Autodesk Fusion 360 part; units mm, degrees
note: some values were not read from the file. Set by a fixed rule: which sketch regions a step uses.
(part 2 of 2)
sketch "Esquisse1 (2)" plane through (0, 0, -35) normal (0, 0, -1) x (1, 0, 0) in component "Component"
  circle A0 centre (290, 50) radius 1.7
  circle A1 centre (10, 10) radius 1.7
  circle A2 centre (80, 90) radius 1.7
  circle A3 centre (150, 10) radius 1.7
  circle A4 centre (220, 90) radius 1.7
  line L0 (282, 72) -> (282, 28)
  arc A5 (272, 18) -> (282, 28) centre (272, 28) ccw
  line L1 (272, 18) -> (28, 18)
  arc A6 (18, 28) -> (28, 18) centre (28, 28) ccw
  line L2 (18, 28) -> (18, 72)
  arc A7 (28, 82) -> (18, 72) centre (28, 72) ccw
  line L3 (28, 82) -> (272, 82)
  arc A8 (282, 72) -> (272, 82) centre (272, 72) ccw
  circle A9 centre (10, 50) radius 1.7
  circle A10 centre (80, 10) radius 1.7
  circle A11 centre (290, 90) radius 1.7
  circle A12 centre (220, 10) radius 1.7
  circle A13 centre (150, 90) radius 1.7
  circle A14 centre (10, 90) radius 1.7
  circle A15 centre (290, 10) radius 1.7
  line L4 (290, 100) -> (10, 100)
  arc A16 (10, 100) -> (0, 90) centre (10, 90) ccw
  line L5 (0, 90) -> (0, 10)
  arc A17 (0, 10) -> (10, 0) centre (10, 10) ccw
  line L6 (10, 0) -> (290, 0)
  arc A18 (290, 0) -> (300, 10) centre (290, 10) ccw
  line L7 (300, 10) -> (300, 90)
  arc A19 (300, 90) -> (290, 100) centre (290, 90) ccw
  line L8 (12.75, 91.587713) -> (10, 93.175426)
  line L9 (10, 93.175426) -> (7.25, 91.587713)
  line L10 (7.25, 91.587713) -> (7.25, 88.412287)
  line L11 (7.25, 88.412287) -> (10, 86.824574)
  line L12 (10, 86.824574) -> (12.75, 88.412287)
  line L13 (12.75, 88.412287) -> (12.75, 91.587713)
  line L14 (80, 93.175426) -> (77.25, 91.587713)
  line L15 (77.25, 91.587713) -> (77.25, 88.412287)
  line L16 (77.25, 88.412287) -> (80, 86.824574)
  line L17 (80, 86.824574) -> (82.75, 88.412287)
  line L18 (82.75, 88.412287) -> (82.75, 91.587713)
  line L19 (82.75, 91.587713) -> (80, 93.175426)
  line L20 (150, 93.175426) -> (147.25, 91.587713)
  line L21 (147.25, 91.587713) -> (147.25, 88.412287)
  line L22 (147.25, 88.412287) -> (150, 86.824574)
  line L23 (150, 86.824574) -> (152.75, 88.412287)
  line L24 (152.75, 88.412287) -> (152.75, 91.587713)
  line L25 (152.75, 91.587713) -> (150, 93.175426)
  line L26 (222.75, 88.412287) -> (222.75, 91.587713)
  line L27 (222.75, 91.587713) -> (220, 93.175426)
  line L28 (220, 93.175426) -> (217.25, 91.587713)
  line L29 (217.25, 91.587713) -> (217.25, 88.412287)
  line L30 (217.25, 88.412287) -> (220, 86.824574)
  line L31 (220, 86.824574) -> (222.75, 88.412287)
  line L32 (290, 86.824574) -> (292.75, 88.412287)
  line L33 (292.75, 88.412287) -> (292.75, 91.587713)
  line L34 (292.75, 91.587713) -> (290, 93.175426)
  line L35 (290, 93.175426) -> (287.25, 91.587713)
  line L36 (287.25, 91.587713) -> (287.25, 88.412287)
  line L37 (287.25, 88.412287) -> (290, 86.824574)
  line L38 (292.75, 51.587713) -> (290, 53.175426)
  line L39 (290, 53.175426) -> (287.25, 51.587713)
  line L40 (287.25, 51.587713) -> (287.25, 48.412287)
  line L41 (287.25, 48.412287) -> (290, 46.824574)
  line L42 (290, 46.824574) -> (292.75, 48.412287)
  line L43 (292.75, 48.412287) -> (292.75, 51.587713)
  line L44 (292.75, 8.412287) -> (292.75, 11.587713)
  line L45 (292.75, 11.587713) -> (290, 13.175426)
  line L46 (290, 13.175426) -> (287.25, 11.587713)
  line L47 (287.25, 11.587713) -> (287.25, 8.412287)
  line L48 (287.25, 8.412287) -> (290, 6.824574)
  line L49 (290, 6.824574) -> (292.75, 8.412287)
  line L50 (222.75, 8.412287) -> (222.75, 11.587713)
  line L51 (222.75, 11.587713) -> (220, 13.175426)
  line L52 (220, 13.175426) -> (217.25, 11.587713)
  line L53 (217.25, 11.587713) -> (217.25, 8.412287)
  line L54 (217.25, 8.412287) -> (220, 6.824574)
  line L55 (220, 6.824574) -> (222.75, 8.412287)
  line L56 (152.75, 8.412287) -> (152.75, 11.587713)
  line L57 (152.75, 11.587713) -> (150, 13.175426)
  line L58 (150, 13.175426) -> (147.25, 11.587713)
  line L59 (147.25, 11.587713) -> (147.25, 8.412287)
  line L60 (147.25, 8.412287) -> (150, 6.824574)
  line L61 (150, 6.824574) -> (152.75, 8.412287)
  line L62 (82.75, 8.412287) -> (82.75, 11.587713)
  line L63 (82.75, 11.587713) -> (80, 13.175426)
  line L64 (80, 13.175426) -> (77.25, 11.587713)
  line L65 (77.25, 11.587713) -> (77.25, 8.412287)
  line L66 (77.25, 8.412287) -> (80, 6.824574)
  line L67 (80, 6.824574) -> (82.75, 8.412287)
  line L68 (12.75, 11.587713) -> (10, 13.175426)
  line L69 (10, 13.175426) -> (7.25, 11.587713)
  line L70 (7.25, 11.587713) -> (7.25, 8.412287)
  line L71 (7.25, 8.412287) -> (10, 6.824574)
  line L72 (10, 6.824574) -> (12.75, 8.412287)
  line L73 (12.75, 8.412287) -> (12.75, 11.587713)
  line L74 (12.75, 48.412287) -> (12.75, 51.587713)
  line L75 (12.75, 51.587713) -> (10, 53.175426)
  line L76 (10, 53.175426) -> (7.25, 51.587713)
  line L77 (7.25, 51.587713) -> (7.25, 48.412287)
  line L78 (7.25, 48.412287) -> (10, 46.824574)
  line L79 (10, 46.824574) -> (12.75, 48.412287)
  circle A20 centre (158.099746, 49.935862) radius 1.7
  circle A21 centre (141.900254, 50.064138) radius 1.7
  line L80 (158.099746, 49.935862) -> (141.900254, 50.064138) construction
  line L81 (0, 90) -> (0, 10) construction
  line L82 (300, 10) -> (300, 90) construction
  point P0 (10, 90)
  point P1 (80, 90)
  point P2 (150, 90)
  point P3 (220, 90)
  point P4 (290, 90)
  point P5 (290, 50)
  point P6 (290, 10)
  point P7 (220, 10)
  point P8 (150, 10)
  point P9 (80, 10)
  point P10 (10, 10)
  point P11 (10, 50)
  point P12 (158.099746, 49.935862)
  point P13 (141.900254, 50.064138)
  point P14 (150, 50)
  point P15 (0, 90)
  point P16 (290, 100)
  dimension "d71" = 5.5
  dimension "d72" = 5.5
  dimension "d73" = 5.5
  dimension "d78" = 5.5
  dimension "d79" = 5.5
  dimension "d80" = 5.5
  dimension "d81" = 5.5
  dimension "d82" = 5.5
  dimension "d83" = 5.5
  dimension "d84" = 5.5
  dimension "d85" = 5.5
  dimension "d86" = 5.5
  dimension "d92" = 3.4
  dimension "d93" = 3.4
  dimension "d94" = 16.2
  dimension "d122" = 150
  dimension "d123" = 300
  dimension "d124" = 100
  dimension "d125" = 50
  constraint coincident P0 A14.centre
  constraint vertical L13
  constraint coincident P1 A2.centre
  constraint coincident P2 A13.centre
  constraint vertical L18
  constraint vertical L24
  constraint coincident P3 A4.centre
  constraint coincident P4 A11.centre
  constraint coincident P5 A0.centre
  constraint coincident P6 A15.centre
  constraint coincident P7 A12.centre
  constraint coincident P8 A3.centre
  constraint coincident P9 A10.centre
  constraint coincident P10 A1.centre
  constraint coincident P11 A9.centre
  constraint vertical L26
  constraint vertical L33
  constraint vertical L43
  constraint vertical L44
  constraint vertical L50
  constraint vertical L56
  constraint vertical L62
  constraint vertical L73
  constraint vertical L74
  constraint midpoint L80 P14
  measures "d78" distance of L26 L29
  measures "d79" distance of L33 L36
  measures "d80" distance of L40 L43
  measures "d81" distance of L44 L47
  measures "d82" distance of L50 L53
  measures "d83" distance of L56 L59
  measures "d84" distance of L62 L65
  measures "d85" distance of L70 L73
  measures "d86" distance of L74 L77
  measures "d92" diameter of A20
  measures "d93" diameter of A21
  measures "d122" distance of P14 L81
  measures "d123" distance of P15 L82
  measures "d124" distance of L6 P16
  measures "d125" distance of L4 P14
extrude "Extrusion4" cut sketch "Esquisse1 (2)" against normal blind 25 contours A0 | A1 | A2 | A3 | A4 | A9 | A10 | A11 | A12 | A13 | A14 | A15 | L8 L9 L10 L11 L12 L13 | L14 L15 L16 L17 L18 L19 | L20 L21 L22 L23 L24 L25 | L26 L27 L28 L29 L30 L31 | L32 L33 L34 L35 L36 L37 | L38 L39 L40 L41 L42 L43 | L44 L45 L46 L47 L48 L49 | L50 L51 L52 L53 L54 L55 | L56 L57 L58 L59 L60 L61 | L62 L63 L64 L65 L66 L67 | L68 L69 L70 L71 L72 L73 | L74 L75 L76 L77 L78 L79 picked at (289.075398, 49.754133) picked at (10.073289, 9.513757) picked at (80.368027, 90.490748) picked at (150.541491, 10.001887) picked at (218.751887, 89.832972) picked at (10.353311, 50.777094) picked at (80.199585, 10.503371) picked at (289.075398, 89.754133) picked at (218.891842, 10.167028) picked at (150.541491, 90.001887) picked at (9.024266, 90.469889) picked at (291.077216, 10.245867) picked at (11.2, 87.921539) picked at (78.8, 87.921539) picked at (151.2, 92.078461) picked at (218.8, 87.921539) picked at (291.2, 87.921539) picked at (291.2, 52.078461) picked at (292.4, 10) picked at (222.4, 10) picked at (151.2, 7.921539) picked at (81.2, 7.921539) picked at (12.4, 10) picked at (12.4, 50) bodies 2 in component "Component"
extrude "Extrusion3" add sketch "Esquisse1 (2)" along normal blind 5 contours L0 A5 L1 A6 L2 A7 L3 A8 | L4 A16 L5 A17 L6 A18 L7 A19 | A20 | A21 picked at (65.400085, 50.021379) picked at (38.416667, 8.804096) picked at (156.991588, 49.768834) picked at (142.441745, 50.066024) bodies 2 in component "Component"
extrude "Extrusion5'" add 1 faces at (55.75, -50.529238, -40) along direction (0, 0, -1) blind 1 on bodies 2 bodies 2 in component "Component"
extrude "Extrusion6'" cut sketch "Esquisse1 (2)" along normal blind 10 contours A20 | A21 picked at (156.991588, 49.768834) picked at (142.441745, 50.066024) bodies 2 in component "Component"
sketch "Esquisse3 (2)" plane through (0, 0, -41) normal (0, 0, -1) x (1, 0, 0) in component "Component"
  circle A0 centre (141.900254, 50.064138) radius 1.7
  circle A1 centre (158.099746, 49.935862) radius 1.7
  line L0 (12.75, 11.587713) -> (12.75, 8.412287)
  line L1 (12.75, 8.412287) -> (10, 6.824574)
  line L2 (10, 6.824574) -> (7.25, 8.412287)
  line L3 (7.25, 8.412287) -> (7.25, 11.587713)
  line L4 (7.25, 11.587713) -> (10, 13.175426)
  line L5 (10, 13.175426) -> (12.75, 11.587713)
  line L6 (12.75, 48.412287) -> (10, 46.824574)
  line L7 (10, 46.824574) -> (7.25, 48.412287)
  line L8 (7.25, 48.412287) -> (7.25, 51.587713)
  line L9 (7.25, 51.587713) -> (10, 53.175426)
  line L10 (10, 53.175426) -> (12.75, 51.587713)
  line L11 (12.75, 51.587713) -> (12.75, 48.412287)
  line L12 (222.75, 88.412287) -> (220, 86.824574)
  line L13 (220, 86.824574) -> (217.25, 88.412287)
  line L14 (217.25, 88.412287) -> (217.25, 91.587713)
  line L15 (217.25, 91.587713) -> (220, 93.175426)
  line L16 (220, 93.175426) -> (222.75, 91.587713)
  line L17 (222.75, 91.587713) -> (222.75, 88.412287)
  line L18 (12.75, 91.587713) -> (12.75, 88.412287)
  line L19 (12.75, 88.412287) -> (10, 86.824574)
  line L20 (10, 86.824574) -> (7.25, 88.412287)
  line L21 (7.25, 88.412287) -> (7.25, 91.587713)
  line L22 (7.25, 91.587713) -> (10, 93.175426)
  line L23 (10, 93.175426) -> (12.75, 91.587713)
  line L24 (150, 93.175426) -> (152.75, 91.587713)
  line L25 (152.75, 91.587713) -> (152.75, 88.412287)
  line L26 (152.75, 88.412287) -> (150, 86.824574)
  line L27 (150, 86.824574) -> (147.25, 88.412287)
  line L28 (147.25, 88.412287) -> (147.25, 91.587713)
  line L29 (147.25, 91.587713) -> (150, 93.175426)
  line L30 (290, 86.824574) -> (287.25, 88.412287)
  line L31 (287.25, 88.412287) -> (287.25, 91.587713)
  line L32 (287.25, 91.587713) -> (290, 93.175426)
  line L33 (290, 93.175426) -> (292.75, 91.587713)
  line L34 (292.75, 91.587713) -> (292.75, 88.412287)
  line L35 (292.75, 88.412287) -> (290, 86.824574)
  line L36 (222.75, 8.412287) -> (220, 6.824574)
  line L37 (220, 6.824574) -> (217.25, 8.412287)
  line L38 (217.25, 8.412287) -> (217.25, 11.587713)
  line L39 (217.25, 11.587713) -> (220, 13.175426)
  line L40 (220, 13.175426) -> (222.75, 11.587713)
  line L41 (222.75, 11.587713) -> (222.75, 8.412287)
  line L42 (80, 93.175426) -> (82.75, 91.587713)
  line L43 (82.75, 91.587713) -> (82.75, 88.412287)
  line L44 (82.75, 88.412287) -> (80, 86.824574)
  line L45 (80, 86.824574) -> (77.25, 88.412287)
  line L46 (77.25, 88.412287) -> (77.25, 91.587713)
  line L47 (77.25, 91.587713) -> (80, 93.175426)
  line L48 (292.75, 51.587713) -> (292.75, 48.412287)
  line L49 (292.75, 48.412287) -> (290, 46.824574)
  line L50 (290, 46.824574) -> (287.25, 48.412287)
  line L51 (287.25, 48.412287) -> (287.25, 51.587713)
  line L52 (287.25, 51.587713) -> (290, 53.175426)
  line L53 (290, 53.175426) -> (292.75, 51.587713)
  line L54 (152.75, 8.412287) -> (150, 6.824574)
  line L55 (150, 6.824574) -> (147.25, 8.412287)
  line L56 (147.25, 8.412287) -> (147.25, 11.587713)
  line L57 (147.25, 11.587713) -> (150, 13.175426)
  line L58 (150, 13.175426) -> (152.75, 11.587713)
  line L59 (152.75, 11.587713) -> (152.75, 8.412287)
  line L60 (82.75, 8.412287) -> (80, 6.824574)
  line L61 (80, 6.824574) -> (77.25, 8.412287)
  line L62 (77.25, 8.412287) -> (77.25, 11.587713)
  line L63 (77.25, 11.587713) -> (80, 13.175426)
  line L64 (80, 13.175426) -> (82.75, 11.587713)
  line L65 (82.75, 11.587713) -> (82.75, 8.412287)
  line L66 (292.75, 8.412287) -> (290, 6.824574)
  line L67 (290, 6.824574) -> (287.25, 8.412287)
  line L68 (287.25, 8.412287) -> (287.25, 11.587713)
  line L69 (287.25, 11.587713) -> (290, 13.175426)
  line L70 (290, 13.175426) -> (292.75, 11.587713)
  line L71 (292.75, 11.587713) -> (292.75, 8.412287)
  arc A2 (300, 90) -> (290, 100) centre (290, 90) ccw
  line L72 (290, 100) -> (10, 100)
  arc A3 (10, 100) -> (0, 90) centre (10, 90) ccw
  line L73 (0, 90) -> (0, 10)
  arc A4 (0, 10) -> (10, 0) centre (10, 10) ccw
  line L74 (10, 0) -> (290, 0)
  arc A5 (290, 0) -> (300, 10) centre (290, 10) ccw
  line L75 (300, 10) -> (300, 90)
  line L76 (155.349746, 51.523575) -> (155.349746, 48.348149)
  line L77 (155.349746, 48.348149) -> (158.099746, 46.760436)
  line L78 (158.099746, 46.760436) -> (160.849746, 48.348149)
  line L79 (160.849746, 48.348149) -> (160.849746, 51.523575)
  line L80 (160.849746, 51.523575) -> (158.099746, 53.111289)
  line L81 (158.099746, 53.111289) -> (155.349746, 51.523575)
  line L82 (139.150254, 51.651851) -> (139.150254, 48.476425)
  line L83 (139.150254, 48.476425) -> (141.900254, 46.888711)
  line L84 (141.900254, 46.888711) -> (144.650254, 48.476425)
  line L85 (144.650254, 48.476425) -> (144.650254, 51.651851)
  line L86 (144.650254, 51.651851) -> (141.900254, 53.239564)
  line L87 (141.900254, 53.239564) -> (139.150254, 51.651851)
  point P0 (158.099746, 49.935862)
  point P1 (141.900254, 50.064138)
  dimension "d101" = 5.5
  dimension "d102" = 5.5
  constraint vertical L76
  constraint vertical L85
  measures "d101" distance of L76 L79
  measures "d102" distance of L82 L85
extrude "Extrusion7" cut sketch "Esquisse3 (2)" against normal blind 3 contours L76 L77 L78 L79 L80 L81 | L82 L83 L84 L85 L86 L87 picked at (160.499746, 49.935862) picked at (140.700254, 52.142599) bodies 2 in component "Component"
ref_plane "Plan de construction1" through (150, -18, -35) normal (0, 0.939693, -0.34202) x (-1, 0, 0) in component "Component"
sketch "Esquisse5" plane through (0, -4.645617, 1.690866) normal (0, 0.939693, -0.34202) x (-1, 0, 0) in component "Component"
  line L0 (-150, -40.861539) -> (-150, -11.731068) construction
  line L1 (-150, -11.731068) -> (-147.25, -12.274098) construction
  line L2 (-147.25, -12.274098) -> (-147.25, -41.404569) construction
  line L3 (-147.25, -41.404569) -> (-150, -40.861539) construction
  line L4 (-152.75, -41.404569) -> (-152.75, -12.274098) construction
  line L5 (-152.75, -12.274098) -> (-150, -11.731068) construction
  line L6 (-150, -11.731068) -> (-150, -40.861539) construction
  line L7 (-150, -40.861539) -> (-152.75, -41.404569) construction
  line L8 (-290, -67.091256) -> (-10, -67.091256) construction
  circle A0 centre (-143.25, -34.045604) radius 3.5
  circle A1 centre (-143.25, -30.545604) radius 3.5
  line L9 (-272, -39.045604) -> (-28, -39.045604)
  line L10 (-146.75, -34.045604) -> (-146.75, -30.545604)
  line L11 (-139.75, -30.545604) -> (-139.75, -34.045604)
  dimension "d106" = 7
  dimension "d107" = 7
  dimension "d108" = 4
  dimension "d110" = 5
  dimension "d120" = 4
  dimension "d121" = 3.5
  constraint vertical L11
  constraint tangent A1 L10
  constraint tangent A1 L11
  constraint tangent A0 L10
  measures "d106" diameter of A1
  measures "d107" diameter of A0
extrude "Extrusion8" cut sketch "Esquisse5" along normal mid plane 40 bodies 2 in component "Component"
sketch "Esquisse6" plane through (0, 0, -35) normal (0, 0, 1) x (-1, 0, 0) in component "Component"
  circle A0 centre (-141.900254, 50.064138) radius 1.7
  circle A1 centre (-158.099746, 49.935862) radius 1.7
  arc A2 (-272, 82) -> (-282, 72) centre (-272, 72) ccw
  line L0 (-282, 72) -> (-282, 28)
  arc A3 (-282, 28) -> (-272, 18) centre (-272, 28) ccw
  line L1 (-272, 18) -> (-28, 18)
  arc A4 (-28, 18) -> (-18, 28) centre (-28, 28) ccw
  line L2 (-18, 28) -> (-18, 72)
  arc A5 (-18, 72) -> (-28, 82) centre (-28, 72) ccw
  line L3 (-28, 82) -> (-272, 82)
  line L4 (-141.900254, 50.064138) -> (-158.099746, 49.935862) construction
  line L5 (-166.5, 44.5) -> (-133.5, 44.5)
  line L6 (-133.5, 44.5) -> (-133.5, 55.5)
  line L7 (-133.5, 55.5) -> (-166.5, 55.5)
  line L8 (-166.5, 55.5) -> (-166.5, 44.5)
  line L9 (-166.5, 44.5) -> (-133.5, 55.5) construction
  line L10 (-133.5, 44.5) -> (-166.5, 55.5) construction
  point P0 (-150, 50)
  dimension "d115" = 33
  dimension "d116" = 11
  constraint horizontal L5
  constraint perpendicular L5 L6
  constraint parallel L5 L7
  constraint parallel L6 L8
  constraint coincident L9 P0
  constraint coincident L10 P0
  constraint midpoint L4 P0
  measures "d115" distance of L6.end L7.end
  measures "d116" distance of L5.end L6.end
extrude "Extrusion9" add sketch "Esquisse6" along normal blind 4 contours L5 L6 L7 L8 picked at (-135.733418, 50.021379) bodies 2 in component "Component"
ref_plane "WorkPlane2" through (150, 0, 0) normal (1, 0, 0) x (0, 1, 0) in component "Component"
component "Component" placed x (1, 0, 0) y (0, 1, 0) z (0, 0, 1) at (0, 0, 0)
equation "d72 = d71"
equation "d73 = d71"
equation "d78 = d71"
equation "d79 = d71"
equation "d80 = d71"
equation "d81 = d71"
equation "d82 = d71"
equation "d83 = d71"
equation "d84 = d71"
equation "d85 = d71"
equation "d86 = d71"
equation "d94 = 8.1 * 2 mm"
equation "d101 = d71"
equation "d102 = d71"
equation "d107 = d106"
equation "d119 = d35 / 2"
equation "d120 = d108"
equation "d122 = d123 / 2"
equation "d125 = d124 / 2"
